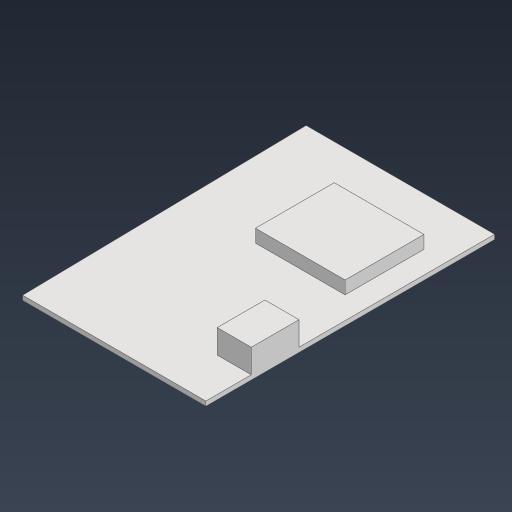
# Autodesk Inventor part: adc
Saved by Autodesk Inventor 2023 (Build 270158000, 158)
## iProperties
Created: 2025-06-15
Part Number: adc
Material: Generic
Document SubType Name: Modeling
Designer: szymo
Density: 1 g/cm^3
Appearance: Default
Author: szymo
Autodesk Inventor part; units mm, degrees
ref_plane "YZ Plane" through (0, 0, 0) normal (1, 0, 0) x (0, 1, 0)
ref_plane "XZ Plane" through (0, 0, 0) normal (0, 1, 0) x (-1, 0, 0)
ref_plane "XY Plane" through (0, 0, 0) normal (0, 0, 1) x (1, 0, 0)
sketch "Sketch1" plane through (0, 0, 0) normal (0, 1, 0) x (-1, 0, 0)
  line L0 (0, 0) -> (24.2, 0)
  line L1 (24.2, 0) -> (24.9, -38.1436)
  line L2 (24.9, -38.1436) -> (0, -38.1436)
  line L3 (0, -38.1436) -> (0, 0)
  dimension "d0" = 38.15
  dimension "d1" = 24.9
  dimension "d2" = 24.2
  constraints: 8 end point, 1 horizontal, 1 parallel, 1 vertical
  measures "d0" distance of L0.end L1.end
  measures "d1" distance of L2.end L1.end
  measures "d2" distance of L0.start L0.end
extrude "Extrusion1" add sketch "Sketch1" along normal blind 0.6
sketch "Sketch2" plane through (0, 0.6, 0) normal (0, 1, 0) x (1, 0, 0)
  line L0 (0, 38.1436) -> (-24.9, 38.1436) projected
  line L1 (-24.9, 38.1436) -> (-24.2, 0) projected
  line L2 (-24.2, 0) -> (0, 0) projected
  line L3 (0, 0) -> (0, 38.1436) projected
  line L4 (0, 6) -> (-4.5, 6)
  line L5 (-4.5, 6) -> (-4.5, 12.3)
  line L6 (-4.5, 12.3) -> (0, 12.3)
  line L7 (0, 12.3) -> (0, 6)
  point P0 (0, 12.3)
  dimension "d5" = 4.5
  dimension "d6" = 6.3
  dimension "d7" = 6
  dimension "d8" = 25.8436
  constraints: 8 end point, 2 parallel, 1 horizontal, 1 perpendicular, 1 point on line
  measures "d5" distance of L5.end L6.end
  measures "d6" distance of L4.end L5.end
  measures "d7" distance between parallel lines of L2 L4
  measures "d8" distance between parallel lines of L0 L6
extrude "Extrusion2" add sketch "Sketch2" along normal blind 3.15 contours L3 L4 L5 L6
sketch "Sketch3" plane through (0, 0.6, 0) normal (0, 1, 0) x (1, 0, 0)
  line L0 (-14.7887, 21.3392) -> (-2.9463, 21.3392)
  line L1 (-2.9463, 21.3392) -> (-2.9463, 31.7514)
  line L2 (-2.9463, 31.7514) -> (-14.7887, 31.7514)
  line L3 (-14.7887, 31.7514) -> (-14.7887, 21.3392)
  point P0 (0, 0)
  constraints: 8 end point, 2 parallel, 1 horizontal, 1 perpendicular
extrude "Extrusion3" add sketch "Sketch3" along normal blind 1.7
sketch "Sketch4" plane through (0, 0, 0) normal (0, -1, 0) x (1, 0, 0)
  line L0 (-17.8896, -8.0503) -> (-7.9992, -8.5103)
  arc A0 (-7.4114, -8.8426) -> (-7.9992, -8.5103) centre (-8.034, -9.258) ccw
  line L1 (-7.4114, -8.8426) -> (-4.5491, -17.8896)
  arc A1 (-4.5491, -18.6308) -> (-4.5491, -17.8896) centre (-5.7203, -18.2602) ccw
  line L2 (-4.5491, -18.6308) -> (-5.7203, -25.9399)
  arc A2 (-5.7203, -25.9399) -> (-5.7203, -25.9399) centre (-3.4138, -26.3096) ccw
  line L3 (-5.7203, -25.9399) -> (-9.7115, -30.1057)
  arc A3 (-10.6571, -30.3612) -> (-9.7115, -30.1057) centre (-10.3961, -29.4497) ccw
  line L4 (-10.6571, -30.3612) -> (-15.5384, -28.2656)
  arc A4 (-16.9185, -26.6044) -> (-15.5384, -28.2656) centre (-14.6016, -26.0835) ccw
  line L5 (-16.9185, -26.6044) -> (-16.9185, -22.4387)
  arc A5 (-16.6885, -21.9531) -> (-16.9185, -22.4387) centre (-16.2909, -22.4387) ccw
  line L6 (-16.6885, -21.9531) -> (-12.7952, -17.8896)
  arc A6 (-13.3329, -16.6318) -> (-12.7952, -17.8896) centre (-11.5884, -16.63) ccw
  line L7 (-13.3329, -16.6318) -> (-16.0354, -15.4715)
  arc A7 (-16.0354, -15.4715) -> (-16.6885, -15.4715) centre (-16.3619, -16.2321) ccw
  line L8 (-16.6885, -15.4715) -> (-18.6774, -15.1528)
  arc A8 (-18.6774, -15.1528) -> (-19.193, -13.8772) centre (-19.9919, -14.9421) ccw
  line L9 (-19.193, -13.8772) -> (-19.193, -11.7599)
  line L10 (-19.193, -11.7599) -> (-17.8896, -8.0503)
  point P0 (0, 0)
  constraints: 22 end point, 18 point on circle, 9 centre point, 7 tangent, 3 parallel, 3 point on line, 1 perpendicular, 1 vertical
extrude "Extrusion4" add sketch "Sketch4" along normal blind 0.9 contours L0 A0 L1 A1 L2 L3 A3 L4 A4 L5 A5 L6 A6 L7 A7 L8 A8 L9 L10
body "Solid1"
